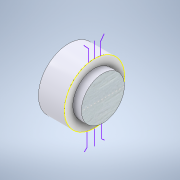
# Autodesk Inventor part: smoke
Saved by Autodesk Inventor 2021 (Build 250183000, 183)
## iProperties
Created: 2021-07-15
Part Number: smoke
Material: Acetal Resin, White
Document SubType Name: Modeling
Designer: HP
Density: 1.425 g/cm^3
Appearance: Smooth - White
Author: HP
Autodesk Inventor part; units mm, degrees
ref_plane "YZ Plane" through (0, 0, 0) normal (1, 0, 0) x (0, 1, 0)
ref_plane "XZ Plane" through (0, 0, 0) normal (0, 1, 0) x (-1, 0, 0)
ref_plane "XY Plane" through (0, 0, 0) normal (0, 0, 1) x (1, 0, 0)
sketch "Sketch1" plane through (0, 0, 0) normal (1, 0, 0) x (0, 1, 0)
  circle A0 centre (0, 0) radius 17.5
  dimension "d0" = 35
  constraints: 1 centre point, 1 coincident
  measures "d0" diameter of A0
extrude "Extrusion1" add sketch "Sketch1" along normal blind 15
sketch "Sketch2" plane through (15, 0, 0) normal (1, 0, 0) x (0, 0, -1)
  circle A0 centre (0, 0) radius 12.5
  circle A1 centre (0, 0) radius 17.5 projected
  line L0 (8.7936, 15.1302) -> (11.8916, 25.206)
  line L1 (11.8916, 25.206) -> (28.1196, 25.206)
  line L2 (-9.2892, 14.8311) -> (-12.729, 25.3334)
  line L3 (-12.729, 25.3334) -> (-30.4043, 25.3334)
  circle A2 centre (0, 0) radius 17.5 projected
  line L4 (-8.5003, -15.2969) -> (-11.9074, -26.8519)
  line L5 (-11.9074, -26.8519) -> (-29.1026, -26.8519)
  line L6 (7.0341, -16.0241) -> (7.2444, -27.3629)
  line L7 (7.2444, -27.3629) -> (28.9362, -28.167)
  dimension "d3" = 25
  constraints: 16 end point, 4 point on circle, 3 horizontal, 1 centre point, 1 coincident
  measures "d3" diameter of A0
extrude "Extrusion2" add sketch "Sketch2" along normal blind 5 contours A0
sketch "Sketch3" plane through (0, 0, 0) normal (0, 1, 0) x (-1, 0, 0)
  point P0 (0, 0)
sketch "Sketch4" plane through (0, 0, 0) normal (0, 0, 1) x (1, 0, 0)
  point P0 (0, 0)
sketch "Sketch5" plane through (15, 0, 0) normal (1, 0, 0) x (0, 0, -1)
  circle A0 centre (0, 0) radius 17.5 projected
  line L0 (0, 17.5) -> (0, 26.5)
  line L1 (-3.3866, 24.2044) -> (-3.3866, 17.1692)
  line L2 (-3.3866, 24.2044) -> (-3.3866, 17.1692)
  line L3 (3.3866, 24.2044) -> (3.3866, 17.1692)
  line L4 (-3.3866, 24.2044) -> (-6.1756, 27.2922)
  line L5 (3.3866, 24.2044) -> (5.6776, 27.2922)
  dimension "d6" = 9
  constraints: 12 end point, 4 vertical, 2 point on circle
  measures "d6" distance of L0.start L0.end
sketch "Sketch6" plane through (15, 0, 0) normal (1, 0, 0) x (0, 0, -1)
  circle A0 centre (0, 0) radius 17.5 projected
  line L0 (0, -17.5) -> (0, -26.5)
  line L1 (4.2832, -25.0802) -> (4.2832, -16.97)
  line L2 (4.2832, -25.0802) -> (5.9397, -26.5)
  line L3 (-4.2832, -25.0802) -> (-4.2832, -16.97)
  line L4 (-4.2832, -25.0802) -> (-5.9397, -26.5)
  dimension "d7" = 9
  constraints: 10 end point, 3 symmetric about line, 2 vertical, 1 vertical alignment, 1 other
  measures "d7" distance of L0.start L0.end
sketch "Sketch7" plane through (0, 0, 0) normal (1, 0, 0) x (0, 1, 0)
  point P0 (0, 0)
body "Solid1"
